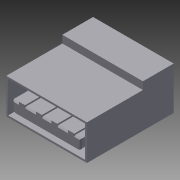
# Autodesk Inventor part: usb host con
Saved by Autodesk Inventor 2012 (Build 160160000, 160)
## iProperties
Created: 2012-02-28
Part Number: usb host con
Material: Default
Document SubType Name: Modeling
Designer: Grailas
Density: 1 g/cm^3
Author: Grailas
Autodesk Inventor part; units mm, degrees
ref_plane "YZ Plane" through (0, 0, 0) normal (1, 0, 0) x (0, 1, 0)
ref_plane "XZ Plane" through (0, 0, 0) normal (0, 1, 0) x (-1, 0, 0)
ref_plane "XY Plane" through (0, 0, 0) normal (0, 0, 1) x (1, 0, 0)
sketch "Sketch1" plane through (0, 0, 0) normal (0, 0, 1) x (1, 0, 0)
  line L0 (-6.55, 7.05) -> (6.55, 7.05)
  line L1 (6.55, 7.05) -> (6.55, -7.05)
  line L2 (6.55, -7.05) -> (-6.55, -7.05)
  line L3 (-6.55, -7.05) -> (-6.55, 7.05)
  point P0 (0, 0)
  point P1 (-6.55, 0)
  point P2 (0, 7.05)
  dimension "d0" = 13.1
  dimension "d1" = 14.1
  constraints: 8 end point, 2 midpoint, 2 parallel, 1 horizontal, 1 horizontal alignment, 1 perpendicular, 1 vertical alignment
  measures "d0" distance of L1.end L2.end
  measures "d1" distance of L0.end L1.end
extrude "Extrusion1" add sketch "Sketch1" along normal blind 5.72
sketch "Sketch2" plane through (0, 0, 5.72) normal (0, 0, 1) x (1, 0, 0)
  line L0 (6.55, 7.05) -> (6.55, -7.05) projected
  line L1 (-6.55, 7.05) -> (6.55, 7.05)
  line L2 (6.55, 7.05) -> (6.55, 2.05)
  line L3 (6.55, 2.05) -> (-6.55, 2.05)
  line L4 (-6.55, 2.05) -> (-6.55, 7.05)
  point P0 (0, 0)
  dimension "d4" = 5
  constraints: 8 end point, 2 parallel, 1 horizontal, 1 perpendicular, 1 point on line
  measures "d4" distance between parallel lines of L1 L3
extrude "Extrusion2" add sketch "Sketch2" along normal blind 1.23
sketch "Sketch3" plane through (-6.55, -7.05, 0) normal (0, -1, 0) x (1, 0, 0)
  line L0 (13.1, 5.72) -> (0, 5.72) projected
  line L1 (0, 0) -> (0, 5.72) projected
  line L2 (13.1, 0) -> (0, 0) projected
  line L3 (13.1, 0) -> (13.1, 5.72) projected
  line L4 (0.3, 5.42) -> (12.8, 5.42)
  line L5 (12.8, 5.42) -> (12.8, 0.3)
  line L6 (12.8, 0.3) -> (0.3, 0.3)
  line L7 (0.3, 0.3) -> (0.3, 5.42)
  line L8 (1, 2.86) -> (12.1, 2.86)
  line L9 (12.1, 2.86) -> (12.1, 1.02)
  line L10 (12.1, 1.02) -> (1, 1.02)
  line L11 (1, 1.02) -> (1, 2.86)
  line L12 (2.05, 2.86) -> (3.05, 2.86)
  line L13 (3.05, 2.86) -> (3.05, 3.11)
  line L14 (3.05, 3.11) -> (2.05, 3.11)
  line L15 (2.05, 3.11) -> (2.05, 2.86)
  line L16 (4.8, 2.86) -> (5.8, 2.86)
  line L17 (5.8, 2.86) -> (5.8, 3.11)
  line L18 (5.8, 3.11) -> (4.8, 3.11)
  line L19 (4.8, 3.11) -> (4.8, 2.86)
  line L20 (7.3, 2.86) -> (8.3, 2.86)
  line L21 (8.3, 2.86) -> (8.3, 3.11)
  line L22 (8.3, 3.11) -> (7.3, 3.11)
  line L23 (7.3, 3.11) -> (7.3, 2.86)
  line L24 (10.05, 2.86) -> (11.05, 2.86)
  line L25 (11.05, 2.86) -> (11.05, 3.11)
  line L26 (11.05, 3.11) -> (10.05, 3.11)
  line L27 (10.05, 3.11) -> (10.05, 2.86)
  point P0 (6.55, 0)
  dimension "d7" = 0.3
  dimension "d9" = 5.72
  dimension "d10" = 5.12
  dimension "d11" = 0.7
  dimension "d13" = 1.84
  dimension "d14" = 0.7
  dimension "d17" = 2.56
  dimension "d20" = 1
  dimension "d21" = 0.25
  dimension "d22" = 1
  dimension "d23" = 1
  dimension "d24" = 1
  dimension "d25" = 0.25
  dimension "d26" = 0.25
  dimension "d27" = 0.25
  dimension "d28" = 1.05
  dimension "d29" = 1.75
  dimension "d30" = 1.5
  dimension "d31" = 1.75
  constraints: 48 end point, 10 parallel, 5 horizontal, 5 perpendicular, 4 point on line, 3 other
  measures "d7" distance between parallel lines of L1 L7
  measures "d9" distance between parallel lines of L2 L0
  measures "d10" distance between parallel lines of L6 L4
  measures "d11" distance between parallel lines of L7 L11
  measures "d13" distance of L10.end L8.start
  measures "d14" distance between parallel lines of L5 L9
  measures "d17" distance between parallel lines of L4 L8
  measures "d20" distance between parallel lines of L13 L15
  measures "d21" distance between parallel lines of L12 L14
  measures "d22" distance between parallel lines of L17 L19
  measures "d23" distance between parallel lines of L21 L23
  measures "d24" distance between parallel lines of L25 L27
  measures "d25" distance between parallel lines of L16 L18
  measures "d26" distance of L22.end L20.start
  measures "d27" distance of L26.end L24.start
  measures "d28" distance between parallel lines of L9 L25
  measures "d29" distance between parallel lines of L21 L27
  measures "d30" distance between parallel lines of L23 L17
  measures "d31" distance between parallel lines of L13 L19
extrude "Extrusion3" cut sketch "Sketch3" against normal blind 10.3 contours L4 L5 L6 L7
fillet "Fillet3" radius 0.64 1 edges at (5.55, -1.9, 1.02)
fillet "Fillet4" radius 0.64 1 edges at (-5.55, -1.9, 1.02)
chamfer "Chamfer1" distance 0.2 angle 45 5 edges at (5.55, -7.05, 2.26) (5.3625, -7.05, 1.2075) (0, -7.05, 1.02) (-5.3625, -7.05, 1.2075) (-5.55, -7.05, 2.26)
chamfer "Chamfer2" distance 0.2 angle 45 1 edges at (4.925, -7.05, 2.86)
chamfer "Chamfer3" distance 0.2 angle 45 1 edges at (2.625, -7.05, 2.86)
chamfer "Chamfer4" distance 0.2 angle 45 1 edges at (0, -7.05, 2.86)
chamfer "Chamfer5" distance 0.2 angle 45 1 edges at (-2.625, -7.05, 2.86)
chamfer "Chamfer6" distance 0.2 angle 45 1 edges at (-4.925, -7.05, 2.86)
body "Solid1"
